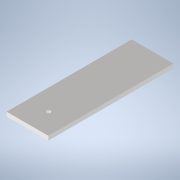
# Autodesk Inventor part: Grundplatte
Saved by Autodesk Inventor 2022 (Build 260153000, 153)
## iProperties
Created: 2022-06-01
Part Number: Grundplatte
Material: Generisch
Document SubType Name: Modeling
Designer: kaebi
Density: 1 g/cm^3
Appearance: Vorgabe
Author: kaebi
Autodesk Inventor part; units mm, degrees
ref_plane "YZ Plane" through (0, 0, 0) normal (1, 0, 0) x (0, 1, 0)
ref_plane "XZ Plane" through (0, 0, 0) normal (0, 1, 0) x (-1, 0, 0)
ref_plane "XY Plane" through (0, 0, 0) normal (0, 0, 1) x (1, 0, 0)
sketch "Skizze1" plane through (0, 0, 0) normal (0, 1, 0) x (-1, 0, 0)
  line L0 (-10, 30) -> (10, 30)
  line L1 (10, 30) -> (10, -30)
  line L2 (10, -30) -> (-10, -30)
  line L3 (-10, -30) -> (-10, 30)
  line L4 (-10, 30) -> (10, -30) construction
  line L5 (10, 30) -> (-10, -30) construction
  circle A0 centre (0, 20) radius 1
  point P0 (0, 0)
  point P1 (0, 0)
  dimension "d0" = 60
  dimension "d1" = 20
  dimension "d2" = 2
  dimension "d3" = 10
  constraints: 12 end point, 3 midpoint, 2 parallel, 1 centre point, 1 horizontal, 1 perpendicular, 1 vertical alignment
  measures "d0" distance of L0.end L1.end
  measures "d1" distance of L1.end L2.end
  measures "d2" diameter of A0
  measures "d3" distance from line of A0.centre L0
extrude "Extrusion1" add sketch "Skizze1" along normal blind 2
